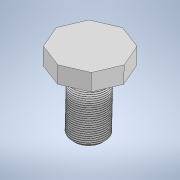
# Autodesk Inventor part: Clamp_Bolt
Saved by Autodesk Inventor 2021 (Build 250183000, 183)
## iProperties
Created: 2021-04-05
Part Number: Clamp_Bolt
Material: Generic
Document SubType Name: Modeling
Designer: Ariel Wolle
Density: 1 g/cm^3
Appearance: Default
Author: Ariel Wolle
Autodesk Inventor part; units mm, degrees
ref_plane "YZ Plane" through (0, 0, 0) normal (1, 0, 0) x (0, 1, 0)
ref_plane "XZ Plane" through (0, 0, 0) normal (0, 1, 0) x (-1, 0, 0)
ref_plane "XY Plane" through (0, 0, 0) normal (0, 0, 1) x (1, 0, 0)
ref_plane "Work Plane3" through (-112.3099, -154.0164, -282.1342) normal (0, -0.9996609, 0.0260402) x (0, -0.0260402, -0.9996609)
sketch "Sketch3" plane through (-112.3099, -154.0164, -282.1342) normal (0, -0.9996609, 0.0260402) x (0, -0.0260402, -0.9996609)
  circle A0 centre (1.463, -34.4711) radius 15
  point P0 (-286.0492, 112.3099)
  dimension "d0" = 30
  constraints: 1 centre point
  measures "d0" diameter of A0
extrude "Extrusion1" add sketch "Sketch3" along normal blind 54
sketch "Sketch4" plane through (-146.781, -154.0545, -283.5967) normal (0, 0.9996609, -0.0260402) x (1, 0, 0)
  circle A0 centre (0, 0) radius 30
  point P0 (146.781, -287.5121)
  dimension "d3" = 60
  constraints: 1 centre point
  measures "d3" diameter of A0
extrude "Extrusion2" add sketch "Sketch4" along normal blind 15
chamfer "Chamfer1" distance 3 angle 45 1 edges at (-146.781, -207.6456, -267.1956)
sketch "Sketch7" plane through (-146.781, -139.0596, -283.9873) normal (0, 0.9996609, -0.0260402) x (1, 0, 0)
  circle A0 centre (0, 0) radius 30
  line L0 (0, 0) -> (-20.6709, -21.742)
  circle A1 centre (0, 0) radius 30 projected
  line L1 (0, 0) -> (-29.9904, -0.7574)
  line L2 (-20.6709, -21.742) -> (-29.9904, -0.7574)
  line L3 (0, 0) -> (0.7574, -29.9904)
  line L4 (0, 0) -> (-20.6709, -21.742)
  line L5 (0.7574, -29.9904) -> (-20.6709, -21.742)
  line L6 (0, 0) -> (21.742, -20.6709)
  line L7 (0, 0) -> (0.7574, -29.9904)
  line L8 (21.742, -20.6709) -> (0.7574, -29.9904)
  line L9 (0, 0) -> (29.9904, 0.7574)
  line L10 (0, 0) -> (21.742, -20.6709)
  line L11 (29.9904, 0.7574) -> (21.742, -20.6709)
  line L12 (0, 0) -> (20.6709, 21.742)
  line L13 (0, 0) -> (29.9904, 0.7574)
  line L14 (20.6709, 21.742) -> (29.9904, 0.7574)
  line L15 (0, 0) -> (-0.7574, 29.9904)
  line L16 (0, 0) -> (20.6709, 21.742)
  line L17 (-0.7574, 29.9904) -> (20.6709, 21.742)
  line L18 (0, 0) -> (-21.742, 20.6709)
  line L19 (0, 0) -> (-0.7574, 29.9904)
  line L20 (-21.742, 20.6709) -> (-0.7574, 29.9904)
  line L21 (0, 0) -> (-29.9904, -0.7574)
  line L22 (0, 0) -> (-21.742, 20.6709)
  line L23 (-29.9904, -0.7574) -> (-21.742, 20.6709)
  point P0 (146.781, -287.5121)
  point P1 (-21.742, 20.6709)
  point P2 (-21.742, 20.6709)
  point P3 (-21.742, 20.6709)
  point P4 (-0.7574, 29.9904)
  point P5 (-0.7574, 29.9904)
  point P6 (-0.7574, 29.9904)
  point P7 (20.6709, 21.742)
  point P8 (20.6709, 21.742)
  point P9 (20.6709, 21.742)
  point P10 (29.9904, 0.7574)
  point P11 (29.9904, 0.7574)
  point P12 (29.9904, 0.7574)
  point P13 (21.742, -20.6709)
  point P14 (21.742, -20.6709)
  point P15 (21.742, -20.6709)
  point P16 (0.7574, -29.9904)
  point P17 (0.7574, -29.9904)
  point P18 (0.7574, -29.9904)
  point P19 (-20.6709, -21.742)
  point P20 (-20.6709, -21.742)
  point P21 (-29.9904, -0.7574)
  point P22 (-29.9904, -0.7574)
  point P23 (-29.9904, -0.7574)
  dimension "d27" = 45
  dimension "d30" = 360
  constraints: 48 end point, 4 point on circle, 3 coincident, 1 centre point, 1 concentric, 55 other
  measures "d27" angle of L1 L0
extrude "Extrusion3" cut sketch "Sketch7" against normal blind 15 contours A0 L11 | L14 A0 | A0 L8 | L17 A0 | A0 L5 | L20 A0 | A0 L2 | A0 L23
ref_plane "Work Plane5" through (-146.781, -154.0545, -283.5967) normal (-0.3592379, 0.024302, 0.9329295) x (0, -0.9996609, 0.0260402)
sketch "Sketch8" plane through (-146.781, -154.0545, -283.5967) normal (-0.3592379, 0.024302, 0.9329295) x (0, -0.9996609, 0.0260402)
  line L0 (51, -15) -> (54, -12) projected
  line L1 (51, -15) -> (50.2777, -11.5098)
  line L2 (51, -15) -> (54, -15) construction
  line L3 (54, -15) -> (54.5627, -13.4994)
  line L4 (54.9373, -13.4994) -> (55.5, -15)
  line L5 (55.5, -15) -> (54, -15)
  line L6 (54.75, -15) -> (54.75, -13) construction
  arc A0 (54.9373, -13.4994) -> (54.5627, -13.4994) centre (54.75, -13.5696) ccw
  line L7 (51, -15) -> (51, 15) projected
  point P0 (-146.6173, 240.2681)
  dimension "d35" = 2
  dimension "d36" = 0.75
  dimension "d37" = 0.2
  dimension "d38" = 3
  constraints: 12 end point, 3 point on line, 2 horizontal, 2 point on circle, 2 tangent, 1 centre point, 1 midpoint, 1 vertical, 1 other
  measures "d35" distance from line of L5 L6.end
  measures "d36" distance from line of L6 L4.end
  measures "d37" radius of A0
  measures "d38" distance from line of L7 L2.end
coil "Coil2" sketch "Sketch8" operation cut axis through (-146.781, -154.0545, -283.5967) along (0, 0.9996609, -0.0260402) pitch 1.7 turns 33.382353 hand right
body "Solid1"
